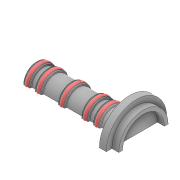
# Autodesk Inventor part: offset_piston
Saved by Autodesk Inventor 2021 (Build 250183000, 183)
## iProperties
Created: 2021-07-12
Part Number: offset_piston
Material: Generic
Document SubType Name: Modeling
Designer: Sihan
Density: 1 g/cm^3
Appearance: Default
Mass: 0.924757 g
Surface Area: 14.8287 cm^2
Volume: 0.924757 cm^3
Author: Sihan
Autodesk Inventor part; units mm, degrees
ref_plane "YZ Plane" through (0, 0, 0) normal (1, 0, 0) x (0, 1, 0)
ref_plane "XZ Plane" through (0, 0, 0) normal (0, 1, 0) x (-1, 0, 0)
ref_plane "XY Plane" through (0, 0, 0) normal (0, 0, 1) x (1, 0, 0)
sketch "Sketch1" plane through (0, 0, 0) normal (0, 0, 1) x (1, 0, 0)
  line L0 (-25.6297, 2.5) -> (-25.6297, 2.91)
  line L1 (-25.6297, 2.91) -> (-24.1297, 2.91)
  line L2 (-24.1297, 2.91) -> (-24.1297, 2.5)
  line L3 (-24.1297, 2.5) -> (-20.6297, 2.5)
  line L4 (-20.6297, 2.5) -> (-20.6297, 2.91)
  line L5 (-20.6297, 2.91) -> (-19.1297, 2.91)
  line L6 (-19.1297, 2.91) -> (-19.1297, 2.5)
  line L7 (-19.1297, 2.5) -> (-18.1297, 2.5)
  line L8 (-18.1297, 2.5) -> (-18.1297, 2.91)
  line L9 (-18.1297, 2.91) -> (-16.6297, 2.91)
  line L10 (-16.6297, 2.91) -> (-16.6297, 2.5)
  line L11 (-13.1297, 6.5) -> (-11.6297, 6.5)
  line L12 (-11.6297, 0) -> (-33.1297, 0)
  line L13 (-11.6297, 6.5) -> (-11.6297, 5.3)
  line L14 (-11.6297, 5.3) -> (-10.1297, 5.3)
  line L15 (-10.1297, 5.3) -> (-10.1297, 4.5)
  line L16 (-10.1297, 4.5) -> (-11.6297, 4.5)
  line L17 (-11.6297, 4.5) -> (-11.6297, 0)
  line L18 (-16.6297, 2.5) -> (-14.1297, 2.5)
  line L19 (-14.1297, 2.5) -> (-14.1297, 4)
  line L20 (-14.1297, 4) -> (-13.1297, 4)
  line L21 (-13.1297, 4) -> (-13.1297, 6.5)
  line L22 (-25.6297, 2.5) -> (-29.1297, 2.5)
  line L23 (-29.1297, 2.5) -> (-29.1297, 2.91)
  line L24 (-29.1297, 2.91) -> (-30.6297, 2.91)
  line L25 (-30.6297, 2.91) -> (-30.6297, 2.5)
  line L26 (-30.6297, 2.5) -> (-31.6297, 2.5)
  line L27 (-31.6297, 2.5) -> (-31.6297, 2.91)
  line L28 (-31.6297, 2.91) -> (-33.1297, 2.91)
  line L29 (-33.1297, 2.91) -> (-33.1297, 0)
  point P0 (0, 0)
  point P1 (-10.1297, 2.5)
  point P2 (-25.6297, 0)
  point P3 (-33.1297, 0.067)
  dimension "d2" = 1.5
  dimension "d3" = 1.5
  dimension "d4" = 1.5
  dimension "d5" = 1.5
  dimension "d9" = 3.5
  dimension "d10" = 1
  dimension "d14" = 6.5
  dimension "d60" = 5.3
  dimension "d61" = 4.5
  dimension "d62" = 1.5
  dimension "d63" = 2.5
  dimension "d64" = 1
  dimension "d65" = 4
  dimension "d95" = 1.5
  dimension "d96" = 3.5
  dimension "d107" = 1
  dimension "d108" = 1.5
  constraints: 60 end point, 18 perpendicular, 10 point on line, 2 horizontal, 2 vertical
  measures "d2" distance of L0.end L1.end
  measures "d3" distance of L4.end L5.end
  measures "d4" distance of L8.end L9.end
  measures "d5" distance of L11.start L11.end
  measures "d9" distance of L2.end L3.end
  measures "d10" distance of L6.end L7.end
  measures "d14" distance between parallel lines of L12 L11
  measures "d60" distance from line of L12.start L14
  measures "d61" distance from line of L12.start L16
  measures "d62" distance between parallel lines of L17 L15
  measures "d63" distance of L10.end L18.end
  measures "d64" distance of L19.end L20.end
  measures "d65" distance between parallel lines of L12 L20
  measures "d95" distance of L23.end L24.end
  measures "d96" distance of L0.start L22.end
  measures "d107" distance of L25.end L26.end
  measures "d108" distance of L27.end L28.end
revolve "Revolution1" add sketch "Sketch1" angle 360 about axis through (-11.6297, 0, 0) along (-1, 0, 0)
chamfer "Chamfer1" distance 0.15 angle 45 7 edges at (-25.6297, -2.91, 0) (-20.6297, -2.91, 0) (-18.1297, -2.91, 0) (-30.6297, -2.91, 0) (-29.1297, -2.91, 0) (-33.1297, -2.91, 0) (-31.6297, -2.91, 0)
chamfer "Chamfer2" distance 0.15 angle 45 3 edges at (-24.1297, -2.91, 0) (-19.1297, -2.91, 0) (-16.6297, -2.91, 0)
sketch "Sketch4" plane through (0, 0, 0) normal (0, 1, 0) x (-1, 0, 0)
  line L0 (17.9797, 2.91) -> (16.7797, 2.91) projected
  arc A0 (16.9297, 2.91) -> (17.8297, 2.91) centre (17.3797, 2.5938) ccw
  line L1 (18.1297, 2.76) -> (18.1297, -2.76) projected
  line L2 (16.6297, -2.76) -> (16.6297, 2.76) projected
  line L3 (20.4797, 2.91) -> (19.2797, 2.91) projected
  arc A1 (19.4297, 2.91) -> (20.3297, 2.91) centre (19.8797, 2.5938) ccw
  line L4 (20.6297, 2.76) -> (20.6297, -2.76) projected
  line L5 (19.1297, -2.76) -> (19.1297, 2.76) projected
  line L6 (25.4797, 2.91) -> (24.2797, 2.91) projected
  arc A2 (24.4297, 2.91) -> (25.3297, 2.91) centre (24.8797, 2.5938) ccw
  line L7 (25.6297, 2.76) -> (25.6297, -2.76) projected
  line L8 (24.1297, -2.76) -> (24.1297, 2.76) projected
  line L9 (30.4797, 2.91) -> (29.2797, 2.91) projected
  arc A3 (29.4297, 2.91) -> (30.3297, 2.91) centre (29.8797, 2.5938) ccw
  line L10 (30.6297, 2.76) -> (30.6297, -2.76) projected
  line L11 (29.1297, -2.76) -> (29.1297, 2.76) projected
  line L12 (32.9797, 2.91) -> (31.7797, 2.91) projected
  arc A4 (31.9297, 2.91) -> (32.8297, 2.91) centre (32.3797, 2.5938) ccw
  line L13 (33.1297, 2.76) -> (33.1297, -2.76) projected
  line L14 (31.6297, -2.76) -> (31.6297, 2.76) projected
  line L15 (39.7557, 0) -> (-6.6259, 0) projected
  point P0 (0, 0)
  dimension "d124" = 0.3
  dimension "d125" = 0.3
  dimension "d126" = 0.55
  dimension "d127" = 0.3
  dimension "d128" = 0.3
  dimension "d129" = 0.55
  dimension "d130" = 0.3
  dimension "d131" = 0.3
  dimension "d133" = 0.55
  dimension "d134" = 0.3
  dimension "d135" = 0.3
  dimension "d136" = 0.55
  dimension "d137" = 0.3
  dimension "d138" = 0.3
  dimension "d139" = 0.55
  constraints: 10 point on circle, 10 point on line, 5 centre point
  measures "d124" distance from line of L1 A0.end
  measures "d125" distance from line of L2 A0.start
  measures "d126" radius of A0
  measures "d127" distance from line of L4 A1.end
  measures "d128" distance from line of L5 A1.start
  measures "d129" radius of A1
  measures "d130" distance from line of L7 A2.end
  measures "d131" distance from line of L8 A2.start
  measures "d133" radius of A2
  measures "d134" distance from line of L10 A3.end
  measures "d135" distance from line of L11 A3.start
  measures "d136" radius of A3
  measures "d137" distance from line of L13 A4.end
  measures "d138" distance from line of L14 A4.start
  measures "d139" radius of A4
revolve "Revolution6" cut sketch "Sketch4" angle 360 about axis through (-10, 0, 0) along (1, 0, 0)
sketch "Sketch5" plane through (0, 0, 0) normal (0, 0, 1) x (1, 0, 0)
  line L0 (-29.2797, 2.91) -> (-29.1297, 2.76) projected
  line L1 (-29.1297, 2.76) -> (-29.1297, 2.5) projected
  line L2 (-29.1297, 2.5) -> (-25.6297, 2.5) projected
  line L3 (-25.6297, 2.5) -> (-25.6297, 2.76) projected
  line L4 (-25.6297, 2.76) -> (-25.4797, 2.91) projected
  line L5 (-25.4797, 2.91) -> (-25.3297, 2.91) projected
  arc A0 (-25.3297, 2.91) -> (-24.4297, 2.91) centre (-24.8797, 2.5938) ccw projected
  line L6 (-24.4297, 2.91) -> (-24.2797, 2.91) projected
  line L7 (-24.2797, 2.91) -> (-24.1297, 2.76) projected
  line L8 (-24.1297, 2.76) -> (-24.1297, 2.5) projected
  line L9 (-24.1297, 2.5) -> (-20.6297, 2.5) projected
  line L10 (-20.6297, 2.5) -> (-20.6297, 2.76) projected
  line L11 (-20.6297, 2.76) -> (-20.4797, 2.91) projected
  line L12 (-20.4797, 2.91) -> (-20.3297, 2.91) projected
  arc A1 (-20.3297, 2.91) -> (-19.4297, 2.91) centre (-19.8797, 2.5938) ccw projected
  line L13 (-19.4297, 2.91) -> (-19.2797, 2.91) projected
  line L14 (-19.2797, 2.91) -> (-19.1297, 2.76) projected
  line L15 (-19.1297, 2.76) -> (-19.1297, 2.5) projected
  line L16 (-19.1297, 2.5) -> (-18.1297, 2.5) projected
  line L17 (-18.1297, 2.5) -> (-18.1297, 2.76) projected
  line L18 (-18.1297, 2.76) -> (-17.9797, 2.91) projected
  line L19 (-17.9797, 2.91) -> (-17.8297, 2.91) projected
  arc A2 (-17.8297, 2.91) -> (-16.9297, 2.91) centre (-17.3797, 2.5938) ccw projected
  line L20 (-16.9297, 2.91) -> (-16.7797, 2.91) projected
  line L21 (-16.7797, 2.91) -> (-16.6297, 2.76) projected
  line L22 (-16.6297, 2.76) -> (-16.6297, 2.5) projected
  line L23 (-16.6297, 2.5) -> (-14.1297, 2.5) projected
  line L24 (-14.1297, 2.5) -> (-14.1297, 4) projected
  line L25 (-14.1297, 4) -> (-13.1297, 4) projected
  line L26 (-13.1297, 4) -> (-13.1297, 6.5) projected
  line L27 (-13.1297, 6.5) -> (-11.6297, 6.5) projected
  line L28 (-11.6297, 6.5) -> (-11.6297, 5.3) projected
  line L29 (-11.6297, 5.3) -> (-10.1297, 5.3) projected
  line L30 (-10.1297, 5.3) -> (-10.1297, 4.5) projected
  line L31 (-10.1297, 4.5) -> (-11.6297, 4.5) projected
  line L32 (-11.6297, 4.5) -> (-11.6297, -4.5) projected
  line L33 (-11.6297, -4.5) -> (-10.1297, -4.5) projected
  line L34 (-10.1297, -4.5) -> (-10.1297, -5.3) projected
  line L35 (-10.1297, -5.3) -> (-11.6297, -5.3) projected
  line L36 (-11.6297, -5.3) -> (-11.6297, -6.5) projected
  line L37 (-11.6297, -6.5) -> (-13.1297, -6.5) projected
  line L38 (-13.1297, -6.5) -> (-13.1297, -4) projected
  line L39 (-13.1297, -4) -> (-14.1297, -4) projected
  line L40 (-14.1297, -4) -> (-14.1297, -2.5) projected
  line L41 (-14.1297, -2.5) -> (-16.6297, -2.5) projected
  line L42 (-16.6297, -2.5) -> (-16.6297, -2.76) projected
  line L43 (-16.6297, -2.76) -> (-16.7797, -2.91) projected
  line L44 (-16.7797, -2.91) -> (-16.9297, -2.91) projected
  arc A3 (-16.9297, -2.91) -> (-17.8297, -2.91) centre (-17.3797, -2.5938) ccw projected
  line L45 (-17.8297, -2.91) -> (-17.9797, -2.91) projected
  line L46 (-17.9797, -2.91) -> (-18.1297, -2.76) projected
  line L47 (-18.1297, -2.76) -> (-18.1297, -2.5) projected
  line L48 (-18.1297, -2.5) -> (-19.1297, -2.5) projected
  line L49 (-19.1297, -2.5) -> (-19.1297, -2.76) projected
  line L50 (-19.1297, -2.76) -> (-19.2797, -2.91) projected
  line L51 (-19.2797, -2.91) -> (-19.4297, -2.91) projected
  arc A4 (-19.4297, -2.91) -> (-20.3297, -2.91) centre (-19.8797, -2.5938) ccw projected
  line L52 (-20.3297, -2.91) -> (-20.4797, -2.91) projected
  line L53 (-20.4797, -2.91) -> (-20.6297, -2.76) projected
  line L54 (-20.6297, -2.76) -> (-20.6297, -2.5) projected
  line L55 (-20.6297, -2.5) -> (-24.1297, -2.5) projected
  line L56 (-24.1297, -2.5) -> (-24.1297, -2.76) projected
  line L57 (-24.1297, -2.76) -> (-24.2797, -2.91) projected
  line L58 (-24.2797, -2.91) -> (-24.4297, -2.91) projected
  arc A5 (-24.4297, -2.91) -> (-25.3297, -2.91) centre (-24.8797, -2.5938) ccw projected
  line L59 (-25.3297, -2.91) -> (-25.4797, -2.91) projected
  line L60 (-25.4797, -2.91) -> (-25.6297, -2.76) projected
  line L61 (-25.6297, -2.76) -> (-25.6297, -2.5) projected
  line L62 (-25.6297, -2.5) -> (-29.1297, -2.5) projected
  line L63 (-29.1297, -2.5) -> (-29.1297, -2.76) projected
  line L64 (-29.1297, -2.76) -> (-29.2797, -2.91) projected
  line L65 (-29.2797, -2.91) -> (-29.4297, -2.91) projected
  arc A6 (-29.4297, -2.91) -> (-30.3297, -2.91) centre (-29.8797, -2.5938) ccw projected
  line L66 (-30.3297, -2.91) -> (-30.4797, -2.91) projected
  line L67 (-30.4797, -2.91) -> (-30.6297, -2.76) projected
  line L68 (-30.6297, -2.76) -> (-30.6297, -2.5) projected
  line L69 (-30.6297, -2.5) -> (-31.6297, -2.5) projected
  line L70 (-31.6297, -2.5) -> (-31.6297, -2.76) projected
  line L71 (-31.6297, -2.76) -> (-31.7797, -2.91) projected
  line L72 (-31.7797, -2.91) -> (-31.9297, -2.91) projected
  arc A7 (-31.9297, -2.91) -> (-32.8297, -2.91) centre (-32.3797, -2.5938) ccw projected
  line L73 (-32.8297, -2.91) -> (-32.9797, -2.91) projected
  line L74 (-32.9797, -2.91) -> (-33.1297, -2.76) projected
  line L75 (-33.1297, -2.76) -> (-33.1297, 2.76) projected
  line L76 (-33.1297, 2.76) -> (-32.9797, 2.91) projected
  line L77 (-32.9797, 2.91) -> (-32.8297, 2.91) projected
  arc A8 (-32.8297, 2.91) -> (-31.9297, 2.91) centre (-32.3797, 2.5938) ccw projected
  line L78 (-31.9297, 2.91) -> (-31.7797, 2.91) projected
  line L79 (-31.7797, 2.91) -> (-31.6297, 2.76) projected
  line L80 (-31.6297, 2.76) -> (-31.6297, 2.5) projected
  line L81 (-31.6297, 2.5) -> (-30.6297, 2.5) projected
  line L82 (-30.6297, 2.5) -> (-30.6297, 2.76) projected
  line L83 (-30.6297, 2.76) -> (-30.4797, 2.91) projected
  line L84 (-30.4797, 2.91) -> (-30.3297, 2.91) projected
  arc A9 (-30.3297, 2.91) -> (-29.4297, 2.91) centre (-29.8797, 2.5938) ccw projected
  line L85 (-29.4297, 2.91) -> (-29.2797, 2.91) projected
  arc A10 (-32.1144, 2.2058) -> (-32.645, 2.2058) centre (-32.3797, 2.5938) ccw
  line L86 (-32.5797, 2.082) -> (-32.5797, 2.0814)
  arc A11 (-32.9297, 2.5938) -> (-31.8297, 2.5938) centre (-32.3797, 2.5938) ccw projected
  line L87 (-32.1797, 2.082) -> (-32.1797, 2.0814)
  arc A12 (-32.5797, 2.082) -> (-32.645, 2.2058) centre (-32.7297, 2.082) ccw
  arc A13 (-32.1144, 2.2058) -> (-32.1797, 2.082) centre (-32.0297, 2.082) ccw
  line L88 (-30.0797, 2.082) -> (-30.0797, 2.0814)
  arc A14 (-30.0797, 2.082) -> (-30.145, 2.2058) centre (-30.2297, 2.082) ccw
  line L89 (-29.6797, 2.082) -> (-29.6797, 2.0814)
  arc A15 (-29.6144, 2.2058) -> (-29.6797, 2.082) centre (-29.5297, 2.082) ccw
  arc A16 (-29.6144, 2.2058) -> (-30.145, 2.2058) centre (-29.8797, 2.5938) ccw
  line L90 (-19.6797, 2.082) -> (-19.6797, 2.0814)
  arc A17 (-19.6144, 2.2058) -> (-19.6797, 2.082) centre (-19.5297, 2.082) ccw
  line L91 (-20.0797, 2.082) -> (-20.0797, 2.0814)
  arc A18 (-20.0797, 2.082) -> (-20.145, 2.2058) centre (-20.2297, 2.082) ccw
  arc A19 (-19.6144, 2.2058) -> (-20.145, 2.2058) centre (-19.8797, 2.5938) ccw
  arc A20 (-17.1144, 2.2058) -> (-17.1797, 2.082) centre (-17.0297, 2.082) ccw
  line L92 (-17.1797, 2.082) -> (-17.1797, 2.0814)
  arc A21 (-17.1144, 2.2058) -> (-17.645, 2.2058) centre (-17.3797, 2.5938) ccw
  line L93 (-17.5797, 2.082) -> (-17.5797, 2.0814)
  arc A22 (-17.5797, 2.082) -> (-17.645, 2.2058) centre (-17.7297, 2.082) ccw
  arc A23 (-24.6144, 2.2058) -> (-24.6797, 2.082) centre (-24.5297, 2.082) ccw
  line L94 (-24.6797, 2.082) -> (-24.6797, 2.0814)
  line L95 (-25.0797, 2.082) -> (-25.0797, 2.0814)
  arc A24 (-25.0797, 2.082) -> (-25.145, 2.2058) centre (-25.2297, 2.082) ccw
  arc A25 (-24.6144, 2.2058) -> (-25.145, 2.2058) centre (-24.8797, 2.5938) ccw
  line L96 (-39.7557, 0) -> (6.6259, 0) projected
  point P0 (0, 0)
  point P1 (-32.5797, 2.1684)
  point P2 (-32.1797, 2.1684)
  point P3 (-29.1297, 2.5)
  point P4 (-29.1297, 2.76)
  point P5 (-30.4297, 2.5938)
  point P6 (-30.6297, 2.76)
  point P7 (-30.4797, 2.91)
  point P8 (-29.2797, 2.91)
  point P9 (-29.3297, 2.5938)
  point P10 (-29.6797, 2.1684)
  point P11 (-30.0797, 2.1684)
  point P12 (-16.6297, 2.76)
  point P13 (-16.6297, 2.5)
  point P14 (-18.1297, 2.5)
  point P15 (-18.1297, 2.76)
  point P16 (-19.1297, 2.5)
  point P17 (-19.1297, 2.76)
  point P18 (-20.6297, 2.76)
  point P19 (-16.7797, 2.91)
  point P20 (-16.9297, 2.91)
  point P21 (-16.9297, 2.91)
  point P22 (-16.8297, 2.5938)
  point P23 (-16.7797, 2.91)
  point P24 (-16.6297, 2.76)
  point P25 (-16.6297, 2.5)
  point P26 (-20.4797, 2.91)
  point P27 (-20.3297, 2.91)
  point P28 (-19.4297, 2.91)
  point P29 (-19.6797, 2.1684)
  point P30 (-20.0797, 2.1684)
  point P31 (-20.4297, 2.5938)
  point P32 (-17.9797, 2.91)
  point P33 (-17.8297, 2.91)
  point P34 (-17.1797, 2.1684)
  point P35 (-17.5797, 2.1684)
  point P36 (-17.8297, 2.91)
  point P37 (-17.9797, 2.91)
  point P38 (-18.1297, 2.76)
  point P39 (-17.9297, 2.5938)
  point P40 (-19.2797, 2.91)
  point P41 (-19.3297, 2.5938)
  point P42 (-24.1297, 2.5)
  point P43 (-24.1297, 2.76)
  point P44 (-25.6297, 2.76)
  point P45 (-24.4297, 2.91)
  point P46 (-24.2797, 2.91)
  point P47 (-25.4797, 2.91)
  point P48 (-25.3297, 2.91)
  point P49 (-25.0797, 2.1684)
  point P50 (-24.6797, 2.1684)
  point P51 (-24.3297, 2.5938)
  point P52 (-25.4297, 2.5938)
  dimension "d141" = 0.2
  dimension "d142" = 0.94
  dimension "d143" = 0.15
  dimension "d144" = 0.15
  dimension "d145" = 0.2
  dimension "d148" = 2.5
  dimension "d155" = 12.5
  dimension "d162" = 7.5
  constraints: 42 point on circle, 20 end point, 15 centre point, 10 point on line, 5 coincident, 4 tangent, 3 horizontal, 1 parallel, 1 vertical, 117 other
  measures "d141" distance from line of L86 A8.centre
  measures "d142" diameter of A10
  measures "d143" radius of A12
  measures "d144" radius of A13
  measures "d145" distance from line of A8.centre L87
  measures "d148" distance of L80.end point (-29.13, 2.5)
  measures "d155" distance of L0.end point (-16.63, 2.76)
  measures "d162" distance of L80.end point (-24.13, 2.5)
revolve "Revolution7" add sketch "Sketch5" angle 360 about axis through (-10, 0, 0) along (1, 0, 0) separate body contours A9 A14 A16 A15 | A24 A25 A23 A0 | A8 A12 A10 A13 | A18 A19 A17 A1 | A22 A21 A20 A2
split "Split1" plane through (0, 0, 0) removes the side toward (0, -1, 0)
split "Split2" plane through (0, 0, 0) removes the side toward (0, -1, 0)
body "Solid1"
body "Solid5"
